Autodesk Inventor part; units mm, degrees
(part 5 of 6)
  line L2000 (-9.6394, -22.1122) -> (-9.6394, -22.3521) construction
  spline S587 degree 2 poles (-9.6394, -22.3521) (-9.6394, -22.5921) (-9.8794, -22.5921) knots 0 0 0 1 1 1
  line L2001 (-9.6394, -22.3521) -> (-9.6394, -22.5921) construction
  line L2002 (-9.6394, -22.5921) -> (-9.8794, -22.5921) construction
  line L2003 (-9.8794, -22.5921) -> (-10.5952, -22.5921)
  spline S588 degree 2 poles (-20.1571, -30.3351) (-19.8611, -30.3351) (-19.4413, -29.9152) (-19.4413, -29.6193) knots 0 0 0 1 2 2 2
  line L2004 (-20.1571, -30.3351) -> (-19.8611, -30.3351) construction
  line L2005 (-19.8611, -30.3351) -> (-19.4413, -29.9152) construction
  line L2006 (-19.4413, -29.9152) -> (-19.4413, -29.6193) construction
  line L2007 (-19.4413, -29.6193) -> (-19.4413, -27.224)
  spline S589 degree 2 poles (-19.4413, -27.224) (-19.4413, -26.928) (-19.8611, -26.5082) (-20.1571, -26.5082) knots 0 0 0 1 2 2 2
  line L2008 (-19.4413, -27.224) -> (-19.4413, -26.928) construction
  line L2009 (-19.4413, -26.928) -> (-19.8611, -26.5082) construction
  line L2010 (-19.8611, -26.5082) -> (-20.1571, -26.5082) construction
  line L2011 (-20.1571, -30.815) -> (-21.5927, -30.815)
  spline S590 degree 2 poles (-21.5927, -30.815) (-21.6886, -30.815) (-21.8326, -30.671) (-21.8326, -30.575) knots 0 0 0 1 2 2 2
  line L2012 (-21.5927, -30.815) -> (-21.6886, -30.815) construction
  line L2013 (-21.6886, -30.815) -> (-21.8326, -30.671) construction
  line L2014 (-21.8326, -30.671) -> (-21.8326, -30.575) construction
  line L2015 (-21.8326, -30.575) -> (-21.8326, -26.2682)
  spline S591 degree 2 poles (-21.8326, -26.2682) (-21.8326, -26.1723) (-21.6886, -26.0283) (-21.5927, -26.0283) knots 0 0 0 1 2 2 2
  line L2016 (-21.8326, -26.2682) -> (-21.8326, -26.1723) construction
  line L2017 (-21.8326, -26.1723) -> (-21.6886, -26.0283) construction
  line L2018 (-21.6886, -26.0283) -> (-21.5927, -26.0283) construction
  line L2019 (-21.5927, -26.0283) -> (-20.1571, -26.0283)
  spline S592 degree 2 poles (-20.1571, -26.0283) (-19.6612, -26.0283) (-18.9614, -26.7321) (-18.9614, -27.224) knots 0 0 0 1 2 2 2
  line L2020 (-20.1571, -26.0283) -> (-19.6612, -26.0283) construction
  line L2021 (-19.6612, -26.0283) -> (-18.9614, -26.7321) construction
  line L2022 (-18.9614, -26.7321) -> (-18.9614, -27.224) construction
  line L2023 (-18.9614, -27.224) -> (-18.9614, -29.6193)
  spline S593 degree 2 poles (-18.9614, -29.6193) (-18.9614, -30.1152) (-19.6612, -30.815) (-20.1571, -30.815) knots 0 0 0 1 2 2 2
  line L2024 (-18.9614, -29.6193) -> (-18.9614, -30.1152) construction
  line L2025 (-18.9614, -30.1152) -> (-19.6612, -30.815) construction
  line L2026 (-19.6612, -30.815) -> (-20.1571, -30.815) construction
  spline S594 degree 2 poles (-22.6464, -34.2509) (-22.4065, -34.2509) (-22.4065, -34.4908) knots 0 0 0 1 1 1
  line L2027 (-22.6464, -34.2509) -> (-22.4065, -34.2509) construction
  line L2028 (-22.4065, -34.2509) -> (-22.4065, -34.4908) construction
  spline S595 degree 2 poles (-22.4065, -34.4908) (-22.4065, -34.7308) (-22.6464, -34.7308) knots 0 0 0 1 1 1
  line L2029 (-22.4065, -34.4908) -> (-22.4065, -34.7308) construction
  line L2030 (-22.4065, -34.7308) -> (-22.6464, -34.7308) construction
  spline S596 degree 2 poles (-24.322, -36.8902) (-24.322, -37.1301) (-24.5619, -37.1301) knots 0 0 0 1 1 1
  line L2031 (-24.322, -36.8902) -> (-24.322, -37.1301) construction
  line L2032 (-24.322, -37.1301) -> (-24.5619, -37.1301) construction
  spline S597 degree 2 poles (-24.5619, -37.1301) (-24.8018, -37.1301) (-24.8018, -36.8902) knots 0 0 0 1 1 1
  line L2033 (-24.5619, -37.1301) -> (-24.8018, -37.1301) construction
  line L2034 (-24.8018, -37.1301) -> (-24.8018, -36.8902) construction
  line L2035 (-24.8018, -36.8902) -> (-24.8018, -32.5834)
  spline S598 degree 2 poles (-24.8018, -32.5834) (-24.8018, -32.3434) (-24.5619, -32.3434) knots 0 0 0 1 1 1
  line L2036 (-24.8018, -32.5834) -> (-24.8018, -32.3434) construction
  line L2037 (-24.8018, -32.3434) -> (-24.5619, -32.3434) construction
  line L2038 (-24.5619, -32.3434) -> (-22.6464, -32.3434)
  spline S599 degree 2 poles (-22.6464, -32.3434) (-22.4065, -32.3434) (-22.4065, -32.5834) knots 0 0 0 1 1 1
  line L2039 (-22.6464, -32.3434) -> (-22.4065, -32.3434) construction
  line L2040 (-22.4065, -32.3434) -> (-22.4065, -32.5834) construction
  spline S600 degree 2 poles (-22.4065, -32.5834) (-22.4065, -32.8233) (-22.6464, -32.8233) knots 0 0 0 1 1 1
  line L2041 (-22.4065, -32.5834) -> (-22.4065, -32.8233) construction
  line L2042 (-22.4065, -32.8233) -> (-22.6464, -32.8233) construction
  line L2043 (10.7293, -22.5371) -> (9.5336, -22.5371)
  spline S601 degree 2 poles (9.5336, -22.5371) (9.1417, -22.5371) (8.5779, -21.9772) (8.5779, -21.5813) knots 0 0 0 1 2 2 2
  line L2044 (9.5336, -22.5371) -> (9.1417, -22.5371) construction
  line L2045 (9.1417, -22.5371) -> (8.5779, -21.9772) construction
  line L2046 (8.5779, -21.9772) -> (8.5779, -21.5813) construction
  line L2047 (8.5779, -21.5813) -> (8.5779, -19.426)
  spline S602 degree 2 poles (8.5779, -19.426) (8.5779, -19.186) (8.8178, -19.186) knots 0 0 0 1 1 1
  line L2048 (8.5779, -19.426) -> (8.5779, -19.186) construction
  line L2049 (8.5779, -19.186) -> (8.8178, -19.186) construction
  spline S603 degree 2 poles (8.8178, -19.186) (9.0578, -19.186) (9.0578, -19.426) knots 0 0 0 1 1 1
  line L2050 (8.8178, -19.186) -> (9.0578, -19.186) construction
  line L2051 (9.0578, -19.186) -> (9.0578, -19.426) construction
  line L2052 (9.0578, -19.426) -> (9.0578, -21.5773)
  spline S604 degree 2 poles (9.0578, -21.5773) (9.0578, -21.7733) (9.3377, -22.0572) (9.5336, -22.0572) knots 0 0 0 1 2 2 2
  line L2053 (9.0578, -21.5773) -> (9.0578, -21.7733) construction
  line L2054 (9.0578, -21.7733) -> (9.3377, -22.0572) construction
  line L2055 (9.3377, -22.0572) -> (9.5336, -22.0572) construction
  spline S605 degree 2 poles (10.4894, -19.426) (10.4894, -19.186) (10.7293, -19.186) knots 0 0 0 1 1 1
  line L2056 (10.4894, -19.426) -> (10.4894, -19.186) construction
  line L2057 (10.4894, -19.186) -> (10.7293, -19.186) construction
  spline S606 degree 2 poles (10.7293, -19.186) (10.9692, -19.186) (10.9692, -19.426) knots 0 0 0 1 1 1
  line L2058 (10.7293, -19.186) -> (10.9692, -19.186) construction
  line L2059 (10.9692, -19.186) -> (10.9692, -19.426) construction
  line L2060 (10.9692, -19.426) -> (10.9692, -22.2971)
  spline S607 degree 2 poles (10.9692, -22.2971) (10.9692, -22.5371) (10.7293, -22.5371) knots 0 0 0 1 1 1
  line L2061 (10.9692, -22.2971) -> (10.9692, -22.5371) construction
  line L2062 (10.9692, -22.5371) -> (10.7293, -22.5371) construction
  spline S608 degree 2 poles (17.6713, -22.5371) (17.4314, -22.5371) (17.4314, -22.2971) knots 0 0 0 1 1 1
  line L2063 (17.6713, -22.5371) -> (17.4314, -22.5371) construction
  line L2064 (17.4314, -22.5371) -> (17.4314, -22.2971) construction
  spline S609 degree 2 poles (16.6716, -21.2374) (16.5797, -21.3694) (16.4757, -21.3694) knots 0 0 0 1 1 1
  line L2065 (16.6716, -21.2374) -> (16.5797, -21.3694) construction
  line L2066 (16.5797, -21.3694) -> (16.4757, -21.3694) construction
  spline S610 degree 2 poles (16.4757, -21.3694) (16.3717, -21.3694) (16.2797, -21.2374) knots 0 0 0 1 1 1
  line L2067 (16.4757, -21.3694) -> (16.3717, -21.3694) construction
  line L2068 (16.3717, -21.3694) -> (16.2797, -21.2374) construction
  spline S611 degree 2 poles (15.52, -22.2971) (15.52, -22.5371) (15.28, -22.5371) knots 0 0 0 1 1 1
  line L2069 (15.52, -22.2971) -> (15.52, -22.5371) construction
  line L2070 (15.52, -22.5371) -> (15.28, -22.5371) construction
  spline S612 degree 2 poles (15.28, -22.5371) (15.0401, -22.5371) (15.0401, -22.2971) knots 0 0 0 1 1 1
  line L2071 (15.28, -22.5371) -> (15.0401, -22.5371) construction
  line L2072 (15.0401, -22.5371) -> (15.0401, -22.2971) construction
  line L2073 (15.0401, -22.2971) -> (15.0401, -19.422)
  spline S613 degree 2 poles (15.0401, -19.422) (15.0401, -19.146) (15.252, -19.146) knots 0 0 0 1 1 1
  line L2074 (15.0401, -19.422) -> (15.0401, -19.146) construction
  line L2075 (15.0401, -19.146) -> (15.252, -19.146) construction
  spline S614 degree 2 poles (15.252, -19.146) (15.376, -19.146) (15.476, -19.286) knots 0 0 0 1 1 1
  line L2076 (15.252, -19.146) -> (15.376, -19.146) construction
  line L2077 (15.376, -19.146) -> (15.476, -19.286) construction
  spline S615 degree 2 poles (17.4754, -19.286) (17.5754, -19.146) (17.6993, -19.146) knots 0 0 0 1 1 1
  line L2078 (17.4754, -19.286) -> (17.5754, -19.146) construction
  line L2079 (17.5754, -19.146) -> (17.6993, -19.146) construction
  spline S616 degree 2 poles (17.6993, -19.146) (17.9113, -19.146) (17.9113, -19.422) knots 0 0 0 1 1 1
  line L2080 (17.6993, -19.146) -> (17.9113, -19.146) construction
  line L2081 (17.9113, -19.146) -> (17.9113, -19.422) construction
  line L2082 (17.9113, -19.422) -> (17.9113, -22.2971)
  spline S617 degree 2 poles (17.9113, -22.2971) (17.9113, -22.5371) (17.6713, -22.5371) knots 0 0 0 1 1 1
  line L2083 (17.9113, -22.2971) -> (17.9113, -22.5371) construction
  line L2084 (17.9113, -22.5371) -> (17.6713, -22.5371) construction
  spline S618 degree 2 poles (7.7252, -27.8713) (7.9211, -27.8713) (8.2011, -27.5874) (8.2011, -27.3914) knots 0 0 0 1 2 2 2
  line L2085 (7.7252, -27.8713) -> (7.9211, -27.8713) construction
  line L2086 (7.9211, -27.8713) -> (8.2011, -27.5874) construction
  line L2087 (8.2011, -27.5874) -> (8.2011, -27.3914) construction
  line L2088 (8.2011, -27.3914) -> (8.2011, -25.9598)
  spline S619 degree 2 poles (8.2011, -25.9598) (8.2011, -25.7639) (7.9211, -25.48) (7.7252, -25.48) knots 0 0 0 1 2 2 2
  line L2089 (8.2011, -25.9598) -> (8.2011, -25.7639) construction
  line L2090 (8.2011, -25.7639) -> (7.9211, -25.48) construction
  line L2091 (7.9211, -25.48) -> (7.7252, -25.48) construction
  line L2092 (7.7252, -25.48) -> (7.2453, -25.48)
  spline S620 degree 2 poles (7.2453, -25.48) (7.0494, -25.48) (6.7695, -25.7639) (6.7695, -25.9598) knots 0 0 0 1 2 2 2
  line L2093 (7.2453, -25.48) -> (7.0494, -25.48) construction
  line L2094 (7.0494, -25.48) -> (6.7695, -25.7639) construction
  line L2095 (6.7695, -25.7639) -> (6.7695, -25.9598) construction
  line L2096 (6.7695, -25.9598) -> (6.7695, -27.3914)
  spline S621 degree 2 poles (6.7695, -27.3914) (6.7695, -27.5874) (7.0494, -27.8713) (7.2453, -27.8713) knots 0 0 0 1 2 2 2
  line L2097 (6.7695, -27.3914) -> (6.7695, -27.5874) construction
  line L2098 (6.7695, -27.5874) -> (7.0494, -27.8713) construction
  line L2099 (7.0494, -27.8713) -> (7.2453, -27.8713) construction
  line L2100 (7.2453, -27.8713) -> (7.7252, -27.8713)
  spline S622 degree 2 poles (6.3616, -23.9764) (6.2736, -23.8884) (6.2736, -23.7804) knots 0 0 0 1 1 1
  line L2101 (6.3616, -23.9764) -> (6.2736, -23.8884) construction
  line L2102 (6.2736, -23.8884) -> (6.2736, -23.7804) construction
  spline S623 degree 2 poles (6.2736, -23.7804) (6.2736, -23.5645) (6.5255, -23.5645) knots 0 0 0 1 1 1
  line L2103 (6.2736, -23.7804) -> (6.2736, -23.5645) construction
  line L2104 (6.2736, -23.5645) -> (6.5255, -23.5645) construction
  line L2105 (6.5255, -23.5645) -> (8.441, -23.5645)
  spline S624 degree 2 poles (8.441, -23.5645) (8.6809, -23.5645) (8.6809, -23.8044) knots 0 0 0 1 1 1
  line L2106 (8.441, -23.5645) -> (8.6809, -23.5645) construction
  line L2107 (8.6809, -23.5645) -> (8.6809, -23.8044) construction
  spline S625 degree 2 poles (8.6809, -23.8044) (8.6809, -24.0444) (8.441, -24.0444) knots 0 0 0 1 1 1
  line L2108 (8.6809, -23.8044) -> (8.6809, -24.0444) construction
  line L2109 (8.6809, -24.0444) -> (8.441, -24.0444) construction
  spline S626 degree 2 poles (8.393, -25.256) (8.433, -25.288) (8.453, -25.332) knots 0 0 0 1 1 1
  line L2110 (8.393, -25.256) -> (8.433, -25.288) construction
  line L2111 (8.433, -25.288) -> (8.453, -25.332) construction
  spline S627 degree 2 poles (8.453, -25.332) (8.6809, -25.5999) (8.6809, -25.9598) knots 0 0 0 1 1 1
  line L2112 (8.453, -25.332) -> (8.6809, -25.5999) construction
  line L2113 (8.6809, -25.5999) -> (8.6809, -25.9598) construction
  line L2114 (8.6809, -25.9598) -> (8.6809, -27.3954)
  spline S628 degree 2 poles (8.6809, -27.3954) (8.6809, -27.7913) (8.1211, -28.3512) (7.7252, -28.3512) knots 0 0 0 1 2 2 2
  line L2115 (8.6809, -27.3954) -> (8.6809, -27.7913) construction
  line L2116 (8.6809, -27.7913) -> (8.1211, -28.3512) construction
  line L2117 (8.1211, -28.3512) -> (7.7252, -28.3512) construction
  line L2118 (7.7252, -28.3512) -> (7.2453, -28.3512)
  spline S629 degree 2 poles (7.2453, -28.3512) (6.8534, -28.3512) (6.2896, -27.7913) (6.2896, -27.3954) knots 0 0 0 1 2 2 2
  line L2119 (7.2453, -28.3512) -> (6.8534, -28.3512) construction
  line L2120 (6.8534, -28.3512) -> (6.2896, -27.7913) construction
  line L2121 (6.2896, -27.7913) -> (6.2896, -27.3954) construction
  line L2122 (6.2896, -27.3954) -> (6.2896, -25.9558)
  spline S630 degree 2 poles (6.2896, -25.9558) (6.2896, -25.5599) (6.8534, -25.0001) (7.2453, -25.0001) knots 0 0 0 1 2 2 2
  line L2123 (6.2896, -25.9558) -> (6.2896, -25.5599) construction
  line L2124 (6.2896, -25.5599) -> (6.8534, -25.0001) construction
  line L2125 (6.8534, -25.0001) -> (7.2453, -25.0001) construction
  spline S631 degree 2 poles (11.0763, -27.8713) (11.2722, -27.8713) (11.5521, -27.5874) (11.5521, -27.3914) knots 0 0 0 1 2 2 2
  line L2126 (11.0763, -27.8713) -> (11.2722, -27.8713) construction
  line L2127 (11.2722, -27.8713) -> (11.5521, -27.5874) construction
  line L2128 (11.5521, -27.5874) -> (11.5521, -27.3914) construction
  spline S632 degree 2 poles (10.5964, -25.48) (10.4004, -25.48) (10.1205, -25.7639) (10.1205, -25.9598) knots 0 0 0 1 2 2 2
  line L2129 (10.5964, -25.48) -> (10.4004, -25.48) construction
  line L2130 (10.4004, -25.48) -> (10.1205, -25.7639) construction
  line L2131 (10.1205, -25.7639) -> (10.1205, -25.9598) construction
  line L2132 (10.1205, -25.9598) -> (10.1205, -27.3914)
  spline S633 degree 2 poles (10.1205, -27.3914) (10.1205, -27.5874) (10.4004, -27.8713) (10.5964, -27.8713) knots 0 0 0 1 2 2 2
  line L2133 (10.1205, -27.3914) -> (10.1205, -27.5874) construction
  line L2134 (10.1205, -27.5874) -> (10.4004, -27.8713) construction
  line L2135 (10.4004, -27.8713) -> (10.5964, -27.8713) construction
  line L2136 (10.5964, -27.8713) -> (11.0763, -27.8713)
  line L2137 (11.0763, -28.3512) -> (10.5964, -28.3512)
  spline S634 degree 2 poles (10.5964, -28.3512) (10.2045, -28.3512) (9.6407, -27.7913) (9.6407, -27.3954) knots 0 0 0 1 2 2 2
  line L2138 (10.5964, -28.3512) -> (10.2045, -28.3512) construction
  line L2139 (10.2045, -28.3512) -> (9.6407, -27.7913) construction
  line L2140 (9.6407, -27.7913) -> (9.6407, -27.3954) construction
  line L2141 (9.6407, -27.3954) -> (9.6407, -25.9558)
  spline S635 degree 2 poles (9.6407, -25.9558) (9.6407, -25.5599) (10.2045, -25.0001) (10.5964, -25.0001) knots 0 0 0 1 2 2 2
  line L2142 (9.6407, -25.9558) -> (9.6407, -25.5599) construction
  line L2143 (9.6407, -25.5599) -> (10.2045, -25.0001) construction
  line L2144 (10.2045, -25.0001) -> (10.5964, -25.0001) construction
  line L2145 (10.5964, -25.0001) -> (11.7921, -25.0001)
  spline S636 degree 2 poles (11.7921, -25.0001) (12.032, -25.0001) (12.032, -25.24) knots 0 0 0 1 1 1
  line L2146 (11.7921, -25.0001) -> (12.032, -25.0001) construction
  line L2147 (12.032, -25.0001) -> (12.032, -25.24) construction
  line L2148 (12.032, -25.24) -> (12.032, -27.3874)
  spline S637 degree 2 poles (12.032, -27.3874) (12.032, -27.7473) (12.3679, -27.8913) knots 0 0 0 1 1 1
  line L2149 (12.032, -27.3874) -> (12.032, -27.7473) construction
  line L2150 (12.032, -27.7473) -> (12.3679, -27.8913) construction
  spline S638 degree 2 poles (12.3679, -27.8913) (12.5159, -27.9513) (12.5159, -28.1032) knots 0 0 0 1 1 1
  line L2151 (12.3679, -27.8913) -> (12.5159, -27.9513) construction
  line L2152 (12.5159, -27.9513) -> (12.5159, -28.1032) construction
  spline S639 degree 2 poles (12.5159, -28.1032) (12.5159, -28.2032) (12.3799, -28.3552) (12.2799, -28.3552) knots 0 0 0 1 2 2 2
  line L2153 (12.5159, -28.1032) -> (12.5159, -28.2032) construction
  line L2154 (12.5159, -28.2032) -> (12.3799, -28.3552) construction
  line L2155 (12.3799, -28.3552) -> (12.2799, -28.3552) construction
  spline S640 degree 2 poles (12.2799, -28.3552) (12.2279, -28.3552) (12.1759, -28.3312) knots 0 0 0 1 1 1
  line L2156 (12.2799, -28.3552) -> (12.2279, -28.3552) construction
  line L2157 (12.2279, -28.3552) -> (12.1759, -28.3312) construction
  spline S641 degree 2 poles (12.1759, -28.3312) (11.936, -28.2272) (11.7881, -28.0352) knots 0 0 0 1 1 1
  line L2158 (12.1759, -28.3312) -> (11.936, -28.2272) construction
  line L2159 (11.936, -28.2272) -> (11.7881, -28.0352) construction
  spline S642 degree 2 poles (11.7881, -28.0352) (11.5001, -28.3512) (11.0763, -28.3512) knots 0 0 0 1 1 1
  line L2160 (11.7881, -28.0352) -> (11.5001, -28.3512) construction
  line L2161 (11.5001, -28.3512) -> (11.0763, -28.3512) construction
  spline S643 degree 2 poles (14.4273, -27.8713) (14.6233, -27.8713) (14.9032, -27.5874) (14.9032, -27.3914) knots 0 0 0 1 2 2 2
  line L2162 (14.4273, -27.8713) -> (14.6233, -27.8713) construction
  line L2163 (14.6233, -27.8713) -> (14.9032, -27.5874) construction
  line L2164 (14.9032, -27.5874) -> (14.9032, -27.3914) construction
  line L2165 (14.9032, -27.3914) -> (14.9032, -25.9598)
  spline S644 degree 2 poles (14.9032, -25.9598) (14.9032, -25.7639) (14.6233, -25.48) (14.4273, -25.48) knots 0 0 0 1 2 2 2
  line L2166 (14.9032, -25.9598) -> (14.9032, -25.7639) construction
  line L2167 (14.9032, -25.7639) -> (14.6233, -25.48) construction
  line L2168 (14.6233, -25.48) -> (14.4273, -25.48) construction
  spline S645 degree 2 poles (13.4716, -29.5468) (13.4716, -29.7867) (13.2317, -29.7867) knots 0 0 0 1 1 1
  line L2169 (13.4716, -29.5468) -> (13.4716, -29.7867) construction
  line L2170 (13.4716, -29.7867) -> (13.2317, -29.7867) construction
  spline S646 degree 2 poles (13.2317, -29.7867) (12.9917, -29.7867) (12.9917, -29.5468) knots 0 0 0 1 1 1
  line L2171 (13.2317, -29.7867) -> (12.9917, -29.7867) construction
  line L2172 (12.9917, -29.7867) -> (12.9917, -29.5468) construction
  line L2173 (12.9917, -29.5468) -> (12.9917, -25.24)
  spline S647 degree 2 poles (12.9917, -25.24) (12.9917, -25.0001) (13.2317, -25.0001) knots 0 0 0 1 1 1
  line L2174 (12.9917, -25.24) -> (12.9917, -25.0001) construction
  line L2175 (12.9917, -25.0001) -> (13.2317, -25.0001) construction
  line L2176 (13.2317, -25.0001) -> (14.4273, -25.0001)
  spline S648 degree 2 poles (14.4273, -25.0001) (14.8232, -25.0001) (15.383, -25.5599) (15.383, -25.9558) knots 0 0 0 1 2 2 2
  line L2177 (14.4273, -25.0001) -> (14.8232, -25.0001) construction
  line L2178 (14.8232, -25.0001) -> (15.383, -25.5599) construction
  line L2179 (15.383, -25.5599) -> (15.383, -25.9558) construction
  line L2180 (15.383, -25.9558) -> (15.383, -27.3954)
  spline S649 degree 2 poles (15.383, -27.3954) (15.383, -27.7913) (14.8232, -28.3512) (14.4273, -28.3512) knots 0 0 0 1 2 2 2
  line L2181 (15.383, -27.3954) -> (15.383, -27.7913) construction
  line L2182 (15.383, -27.7913) -> (14.8232, -28.3512) construction
  line L2183 (14.8232, -28.3512) -> (14.4273, -28.3512) construction
  spline S650 degree 2 poles (7.6622, -35.058) (7.8581, -35.058) (8.138, -34.7741) (8.138, -34.5782) knots 0 0 0 1 2 2 2
  line L2184 (7.6622, -35.058) -> (7.8581, -35.058) construction
  line L2185 (7.8581, -35.058) -> (8.138, -34.7741) construction
  line L2186 (8.138, -34.7741) -> (8.138, -34.5782) construction
  spline S651 degree 2 poles (7.1823, -32.6667) (6.9863, -32.6667) (6.7064, -32.9506) (6.7064, -33.1466) knots 0 0 0 1 2 2 2
  line L2187 (7.1823, -32.6667) -> (6.9863, -32.6667) construction
  line L2188 (6.9863, -32.6667) -> (6.7064, -32.9506) construction
  line L2189 (6.7064, -32.9506) -> (6.7064, -33.1466) construction
  line L2190 (6.7064, -33.1466) -> (6.7064, -34.5782)
  spline S652 degree 2 poles (6.7064, -34.5782) (6.7064, -34.7741) (6.9863, -35.058) (7.1823, -35.058) knots 0 0 0 1 2 2 2
  line L2191 (6.7064, -34.5782) -> (6.7064, -34.7741) construction
  line L2192 (6.7064, -34.7741) -> (6.9863, -35.058) construction
  line L2193 (6.9863, -35.058) -> (7.1823, -35.058) construction
  line L2194 (7.1823, -35.058) -> (7.6622, -35.058)
  line L2195 (7.6622, -35.5379) -> (7.1823, -35.5379)
  spline S653 degree 2 poles (7.1823, -35.5379) (6.7904, -35.5379) (6.2266, -34.9781) (6.2266, -34.5822) knots 0 0 0 1 2 2 2
  line L2196 (7.1823, -35.5379) -> (6.7904, -35.5379) construction
  line L2197 (6.7904, -35.5379) -> (6.2266, -34.9781) construction
  line L2198 (6.2266, -34.9781) -> (6.2266, -34.5822) construction
  line L2199 (6.2266, -34.5822) -> (6.2266, -33.1426)
  spline S654 degree 2 poles (6.2266, -33.1426) (6.2266, -32.7467) (6.7904, -32.1868) (7.1823, -32.1868) knots 0 0 0 1 2 2 2
  line L2200 (6.2266, -33.1426) -> (6.2266, -32.7467) construction
  line L2201 (6.2266, -32.7467) -> (6.7904, -32.1868) construction
  line L2202 (6.7904, -32.1868) -> (7.1823, -32.1868) construction
  line L2203 (7.1823, -32.1868) -> (8.3779, -32.1868)
  spline S655 degree 2 poles (8.3779, -32.1868) (8.6179, -32.1868) (8.6179, -32.4268) knots 0 0 0 1 1 1
  line L2204 (8.3779, -32.1868) -> (8.6179, -32.1868) construction
  line L2205 (8.6179, -32.1868) -> (8.6179, -32.4268) construction
  line L2206 (8.6179, -32.4268) -> (8.6179, -34.5742)
  spline S656 degree 2 poles (8.6179, -34.5742) (8.6179, -34.9341) (8.9538, -35.078) knots 0 0 0 1 1 1
  line L2207 (8.6179, -34.5742) -> (8.6179, -34.9341) construction
  line L2208 (8.6179, -34.9341) -> (8.9538, -35.078) construction
  spline S657 degree 2 poles (8.9538, -35.078) (9.1017, -35.138) (9.1017, -35.29) knots 0 0 0 1 1 1
  line L2209 (8.9538, -35.078) -> (9.1017, -35.138) construction
  line L2210 (9.1017, -35.138) -> (9.1017, -35.29) construction
  spline S658 degree 2 poles (9.1017, -35.29) (9.1017, -35.3899) (8.9658, -35.5419) (8.8658, -35.5419) knots 0 0 0 1 2 2 2
  line L2211 (9.1017, -35.29) -> (9.1017, -35.3899) construction
  line L2212 (9.1017, -35.3899) -> (8.9658, -35.5419) construction
  line L2213 (8.9658, -35.5419) -> (8.8658, -35.5419) construction
  spline S659 degree 2 poles (8.8658, -35.5419) (8.8138, -35.5419) (8.7618, -35.5179) knots 0 0 0 1 1 1
  line L2214 (8.8658, -35.5419) -> (8.8138, -35.5419) construction
  line L2215 (8.8138, -35.5419) -> (8.7618, -35.5179) construction
  spline S660 degree 2 poles (8.7618, -35.5179) (8.5219, -35.4139) (8.374, -35.222) knots 0 0 0 1 1 1
  line L2216 (8.7618, -35.5179) -> (8.5219, -35.4139) construction
  line L2217 (8.5219, -35.4139) -> (8.374, -35.222) construction
  spline S661 degree 2 poles (8.374, -35.222) (8.086, -35.5379) (7.6622, -35.5379) knots 0 0 0 1 1 1
  line L2218 (8.374, -35.222) -> (8.086, -35.5379) construction
  line L2219 (8.086, -35.5379) -> (7.6622, -35.5379) construction
  line L2220 (10.0095, -34.5342) -> (10.0095, -35.298)
  spline S662 degree 2 poles (10.0095, -35.298) (10.0095, -35.5379) (9.7696, -35.5379) knots 0 0 0 1 1 1
  line L2221 (10.0095, -35.298) -> (10.0095, -35.5379) construction
  line L2222 (10.0095, -35.5379) -> (9.7696, -35.5379) construction
  spline S663 degree 2 poles (9.7696, -35.5379) (9.5296, -35.5379) (9.5296, -35.298) knots 0 0 0 1 1 1
  line L2223 (9.7696, -35.5379) -> (9.5296, -35.5379) construction
  line L2224 (9.5296, -35.5379) -> (9.5296, -35.298) construction
  line L2225 (9.5296, -35.298) -> (9.5296, -32.4268)
  spline S664 degree 2 poles (9.5296, -32.4268) (9.5296, -32.1868) (9.7696, -32.1868) knots 0 0 0 1 1 1
  line L2226 (9.5296, -32.4268) -> (9.5296, -32.1868) construction
  line L2227 (9.5296, -32.1868) -> (9.7696, -32.1868) construction
  spline S665 degree 2 poles (9.7696, -32.1868) (10.0095, -32.1868) (10.0095, -32.4268) knots 0 0 0 1 1 1
  line L2228 (9.7696, -32.1868) -> (10.0095, -32.1868) construction
  line L2229 (10.0095, -32.1868) -> (10.0095, -32.4268) construction
  spline S666 degree 2 poles (11.5291, -32.2428) (11.593, -32.1708) (11.681, -32.1708) knots 0 0 0 1 1 1
  line L2230 (11.5291, -32.2428) -> (11.593, -32.1708) construction
  line L2231 (11.593, -32.1708) -> (11.681, -32.1708) construction
  spline S667 degree 2 poles (11.681, -32.1708) (11.777, -32.1708) (11.921, -32.3268) (11.921, -32.4308) knots 0 0 0 1 2 2 2
  line L2232 (11.681, -32.1708) -> (11.777, -32.1708) construction
  line L2233 (11.777, -32.1708) -> (11.921, -32.3268) construction
  line L2234 (11.921, -32.3268) -> (11.921, -32.4308) construction
  spline S668 degree 2 poles (11.921, -32.4308) (11.921, -32.5307) (11.845, -32.6067) knots 0 0 0 1 1 1
  line L2235 (11.921, -32.4308) -> (11.921, -32.5307) construction
  line L2236 (11.921, -32.5307) -> (11.845, -32.6067) construction
  spline S669 degree 2 poles (11.869, -35.142) (11.921, -35.222) (11.921, -35.302) knots 0 0 0 1 1 1
  line L2237 (11.869, -35.142) -> (11.921, -35.222) construction
  line L2238 (11.921, -35.222) -> (11.921, -35.302) construction
  spline S670 degree 2 poles (11.921, -35.302) (11.921, -35.4019) (11.765, -35.5459) (11.677, -35.5459) knots 0 0 0 1 2 2 2
  line L2239 (11.921, -35.302) -> (11.921, -35.4019) construction
  line L2240 (11.921, -35.4019) -> (11.765, -35.5459) construction
  line L2241 (11.765, -35.5459) -> (11.677, -35.5459) construction
  spline S671 degree 2 poles (11.677, -35.5459) (11.5651, -35.5459) (11.5051, -35.4499) knots 0 0 0 1 1 1
  line L2242 (11.677, -35.5459) -> (11.5651, -35.5459) construction
  line L2243 (11.5651, -35.5459) -> (11.5051, -35.4499) construction
  line L2244 (11.5051, -35.4499) -> (10.5453, -33.9703)
  spline S672 degree 2 poles (10.5453, -33.9703) (10.4014, -34.1223) (10.0095, -34.5342) knots 0 0 0 1 1 1
  line L2245 (10.5453, -33.9703) -> (10.4014, -34.1223) construction
  line L2246 (10.4014, -34.1223) -> (10.0095, -34.5342) construction
  spline S673 degree 2 poles (-21.2583, -43.6884) (-21.2583, -43.4485) (-21.0184, -43.4485) knots 0 0 0 1 1 1
  line L2247 (-21.2583, -43.6884) -> (-21.2583, -43.4485) construction
  line L2248 (-21.2583, -43.4485) -> (-21.0184, -43.4485) construction
  spline S674 degree 2 poles (-21.0184, -43.4485) (-20.7785, -43.4485) (-20.7785, -43.6884) knots 0 0 0 1 1 1
  line L2249 (-21.0184, -43.4485) -> (-20.7785, -43.4485) construction
  line L2250 (-20.7785, -43.4485) -> (-20.7785, -43.6884) construction
  line L2251 (-20.7785, -43.6884) -> (-20.7785, -46.5596)
  spline S675 degree 2 poles (-20.7785, -46.5596) (-20.7785, -46.7995) (-21.0184, -46.7995) knots 0 0 0 1 1 1
  line L2252 (-20.7785, -46.5596) -> (-20.7785, -46.7995) construction
  line L2253 (-20.7785, -46.7995) -> (-21.0184, -46.7995) construction
  spline S676 degree 2 poles (-21.0184, -46.7995) (-21.2583, -46.7995) (-21.2583, -46.5596) knots 0 0 0 1 1 1
  line L2254 (-21.0184, -46.7995) -> (-21.2583, -46.7995) construction
  line L2255 (-21.2583, -46.7995) -> (-21.2583, -46.5596) construction
  spline S677 degree 2 poles (-22.6899, -46.5596) (-22.6899, -46.7995) (-22.9299, -46.7995) knots 0 0 0 1 1 1
  line L2256 (-22.6899, -46.5596) -> (-22.6899, -46.7995) construction
  line L2257 (-22.6899, -46.7995) -> (-22.9299, -46.7995) construction
  spline S678 degree 2 poles (-22.9299, -46.7995) (-23.1698, -46.7995) (-23.1698, -46.5596) knots 0 0 0 1 1 1
  line L2258 (-22.9299, -46.7995) -> (-23.1698, -46.7995) construction
  line L2259 (-23.1698, -46.7995) -> (-23.1698, -46.5596) construction
  line L2260 (-23.1698, -46.5596) -> (-23.1698, -43.6884)
  spline S679 degree 2 poles (-23.1698, -43.6884) (-23.1698, -43.4485) (-22.9299, -43.4485) knots 0 0 0 1 1 1
  line L2261 (-23.1698, -43.6884) -> (-23.1698, -43.4485) construction
  line L2262 (-23.1698, -43.4485) -> (-22.9299, -43.4485) construction
  spline S680 degree 2 poles (-22.9299, -43.4485) (-22.6899, -43.4485) (-22.6899, -43.6884) knots 0 0 0 1 1 1
  line L2263 (-22.9299, -43.4485) -> (-22.6899, -43.4485) construction
  line L2264 (-22.6899, -43.4485) -> (-22.6899, -43.6884) construction
  spline S681 degree 2 poles (-11.681, -46.3197) (-11.4851, -46.3197) (-11.2052, -46.0357) (-11.2052, -45.8398) knots 0 0 0 1 2 2 2
  line L2265 (-11.681, -46.3197) -> (-11.4851, -46.3197) construction
  line L2266 (-11.4851, -46.3197) -> (-11.2052, -46.0357) construction
  line L2267 (-11.2052, -46.0357) -> (-11.2052, -45.8398) construction
  line L2268 (-11.2052, -45.8398) -> (-11.2052, -44.4082)
  spline S682 degree 2 poles (-11.2052, -44.4082) (-11.2052, -44.2123) (-11.4851, -43.9283) (-11.681, -43.9283) knots 0 0 0 1 2 2 2
  line L2269 (-11.2052, -44.4082) -> (-11.2052, -44.2123) construction
  line L2270 (-11.2052, -44.2123) -> (-11.4851, -43.9283) construction
  line L2271 (-11.4851, -43.9283) -> (-11.681, -43.9283) construction
  spline S683 degree 2 poles (-12.6368, -47.9952) (-12.6368, -48.2351) (-12.8767, -48.2351) knots 0 0 0 1 1 1
  line L2272 (-12.6368, -47.9952) -> (-12.6368, -48.2351) construction
  line L2273 (-12.6368, -48.2351) -> (-12.8767, -48.2351) construction
  spline S684 degree 2 poles (-12.8767, -48.2351) (-13.1166, -48.2351) (-13.1166, -47.9952) knots 0 0 0 1 1 1
  line L2274 (-12.8767, -48.2351) -> (-13.1166, -48.2351) construction
  line L2275 (-13.1166, -48.2351) -> (-13.1166, -47.9952) construction
  line L2276 (-13.1166, -47.9952) -> (-13.1166, -43.6884)
  spline S685 degree 2 poles (-13.1166, -43.6884) (-13.1166, -43.4485) (-12.8767, -43.4485) knots 0 0 0 1 1 1
  line L2277 (-13.1166, -43.6884) -> (-13.1166, -43.4485) construction
  line L2278 (-13.1166, -43.4485) -> (-12.8767, -43.4485) construction
  line L2279 (-12.8767, -43.4485) -> (-11.681, -43.4485)
  spline S686 degree 2 poles (-11.681, -43.4485) (-11.2852, -43.4485) (-10.7253, -44.0083) (-10.7253, -44.4042) knots 0 0 0 1 2 2 2
  line L2280 (-11.681, -43.4485) -> (-11.2852, -43.4485) construction
  line L2281 (-11.2852, -43.4485) -> (-10.7253, -44.0083) construction
  line L2282 (-10.7253, -44.0083) -> (-10.7253, -44.4042) construction
  line L2283 (-10.7253, -44.4042) -> (-10.7253, -45.8438)
  spline S687 degree 2 poles (-10.7253, -45.8438) (-10.7253, -46.2397) (-11.2852, -46.7995) (-11.681, -46.7995) knots 0 0 0 1 2 2 2
  line L2284 (-10.7253, -45.8438) -> (-10.7253, -46.2397) construction
  line L2285 (-10.7253, -46.2397) -> (-11.2852, -46.7995) construction
  line L2286 (-11.2852, -46.7995) -> (-11.681, -46.7995) construction
  spline S688 degree 2 poles (-8.33, -46.3197) (-8.134, -46.3197) (-7.8541, -46.0357) (-7.8541, -45.8398) knots 0 0 0 1 2 2 2
  line L2287 (-8.33, -46.3197) -> (-8.134, -46.3197) construction
  line L2288 (-8.134, -46.3197) -> (-7.8541, -46.0357) construction
  line L2289 (-7.8541, -46.0357) -> (-7.8541, -45.8398) construction
  spline S689 degree 2 poles (-8.8099, -43.9283) (-9.0058, -43.9283) (-9.2857, -44.2123) (-9.2857, -44.4082) knots 0 0 0 1 2 2 2
  line L2290 (-8.8099, -43.9283) -> (-9.0058, -43.9283) construction
  line L2291 (-9.0058, -43.9283) -> (-9.2857, -44.2123) construction
  line L2292 (-9.2857, -44.2123) -> (-9.2857, -44.4082) construction
  line L2293 (-9.2857, -44.4082) -> (-9.2857, -45.8398)
  spline S690 degree 2 poles (-9.2857, -45.8398) (-9.2857, -46.0357) (-9.0058, -46.3197) (-8.8099, -46.3197) knots 0 0 0 1 2 2 2
  line L2294 (-9.2857, -45.8398) -> (-9.2857, -46.0357) construction
  line L2295 (-9.2857, -46.0357) -> (-9.0058, -46.3197) construction
  line L2296 (-9.0058, -46.3197) -> (-8.8099, -46.3197) construction
  line L2297 (-8.8099, -46.3197) -> (-8.33, -46.3197)
  line L2298 (-8.33, -46.7995) -> (-8.8099, -46.7995)
  spline S691 degree 2 poles (-8.8099, -46.7995) (-9.2017, -46.7995) (-9.7656, -46.2397) (-9.7656, -45.8438) knots 0 0 0 1 2 2 2
  line L2299 (-8.8099, -46.7995) -> (-9.2017, -46.7995) construction
  line L2300 (-9.2017, -46.7995) -> (-9.7656, -46.2397) construction
  line L2301 (-9.7656, -46.2397) -> (-9.7656, -45.8438) construction
  line L2302 (-9.7656, -45.8438) -> (-9.7656, -44.4042)
  spline S692 degree 2 poles (-9.7656, -44.4042) (-9.7656, -44.0083) (-9.2017, -43.4485) (-8.8099, -43.4485) knots 0 0 0 1 2 2 2
  line L2303 (-9.7656, -44.4042) -> (-9.7656, -44.0083) construction
  line L2304 (-9.7656, -44.0083) -> (-9.2017, -43.4485) construction
  line L2305 (-9.2017, -43.4485) -> (-8.8099, -43.4485) construction
  line L2306 (-8.8099, -43.4485) -> (-7.6142, -43.4485)
  spline S693 degree 2 poles (-7.6142, -43.4485) (-7.3743, -43.4485) (-7.3743, -43.6884) knots 0 0 0 1 1 1
  line L2307 (-7.6142, -43.4485) -> (-7.3743, -43.4485) construction
  line L2308 (-7.3743, -43.4485) -> (-7.3743, -43.6884) construction
  line L2309 (-7.3743, -43.6884) -> (-7.3743, -45.8358)
  spline S694 degree 2 poles (-7.3743, -45.8358) (-7.3743, -46.1957) (-7.0384, -46.3397) knots 0 0 0 1 1 1
  line L2310 (-7.3743, -45.8358) -> (-7.3743, -46.1957) construction
  line L2311 (-7.3743, -46.1957) -> (-7.0384, -46.3397) construction
  spline S695 degree 2 poles (-7.0384, -46.3397) (-6.8904, -46.3996) (-6.8904, -46.5516) knots 0 0 0 1 1 1
  line L2312 (-7.0384, -46.3397) -> (-6.8904, -46.3996) construction
  line L2313 (-6.8904, -46.3996) -> (-6.8904, -46.5516) construction
  spline S696 degree 2 poles (-6.8904, -46.5516) (-6.8904, -46.6516) (-7.0264, -46.8035) (-7.1263, -46.8035) knots 0 0 0 1 2 2 2
  line L2314 (-6.8904, -46.5516) -> (-6.8904, -46.6516) construction
  line L2315 (-6.8904, -46.6516) -> (-7.0264, -46.8035) construction
  line L2316 (-7.0264, -46.8035) -> (-7.1263, -46.8035) construction
  spline S697 degree 2 poles (-7.1263, -46.8035) (-7.1783, -46.8035) (-7.2303, -46.7795) knots 0 0 0 1 1 1
  line L2317 (-7.1263, -46.8035) -> (-7.1783, -46.8035) construction
  line L2318 (-7.1783, -46.8035) -> (-7.2303, -46.7795) construction
  spline S698 degree 2 poles (-7.2303, -46.7795) (-7.4702, -46.6756) (-7.6182, -46.4836) knots 0 0 0 1 1 1
  line L2319 (-7.2303, -46.7795) -> (-7.4702, -46.6756) construction
  line L2320 (-7.4702, -46.6756) -> (-7.6182, -46.4836) construction
  spline S699 degree 2 poles (-7.6182, -46.4836) (-7.9061, -46.7995) (-8.33, -46.7995) knots 0 0 0 1 1 1
  line L2321 (-7.6182, -46.4836) -> (-7.9061, -46.7995) construction
  line L2322 (-7.9061, -46.7995) -> (-8.33, -46.7995) construction
  line L2323 (-5.9347, -42.8726) -> (-5.9347, -43.6164)
  spline S700 degree 2 poles (-5.9347, -43.6164) (-5.7467, -43.4965) (-5.4588, -43.2845) knots 0 0 0 1 1 1
  line L2324 (-5.9347, -43.6164) -> (-5.7467, -43.4965) construction
  line L2325 (-5.7467, -43.4965) -> (-5.4588, -43.2845) construction
  spline S701 degree 2 poles (-5.4588, -43.2845) (-5.1709, -43.0526) (-5.1709, -42.8726) knots 0 0 0 1 1 1
  line L2326 (-5.4588, -43.2845) -> (-5.1709, -43.0526) construction
  line L2327 (-5.1709, -43.0526) -> (-5.1709, -42.8726) construction
  spline S702 degree 2 poles (-5.1709, -42.8726) (-5.1709, -42.6887) (-5.2908, -42.5847) knots 0 0 0 1 1 1
  line L2328 (-5.1709, -42.8726) -> (-5.1709, -42.6887) construction
  line L2329 (-5.1709, -42.6887) -> (-5.2908, -42.5847) construction
  spline S703 degree 2 poles (-5.2908, -42.5847) (-5.3988, -42.4927) (-5.5508, -42.4927) knots 0 0 0 1 1 1
  line L2330 (-5.2908, -42.5847) -> (-5.3988, -42.4927) construction
  line L2331 (-5.3988, -42.4927) -> (-5.5508, -42.4927) construction
  spline S704 degree 2 poles (-5.5508, -42.4927) (-5.7107, -42.4927) (-5.8147, -42.5847) knots 0 0 0 1 1 1
  line L2332 (-5.5508, -42.4927) -> (-5.7107, -42.4927) construction
  line L2333 (-5.7107, -42.4927) -> (-5.8147, -42.5847) construction
  spline S705 degree 2 poles (-5.8147, -42.5847) (-5.9347, -42.6887) (-5.9347, -42.8726) knots 0 0 0 1 1 1
  line L2334 (-5.8147, -42.5847) -> (-5.9347, -42.6887) construction
  line L2335 (-5.9347, -42.6887) -> (-5.9347, -42.8726) construction
  spline S706 degree 2 poles (-4.9789, -46.3197) (-4.783, -46.3197) (-4.5031, -46.0357) (-4.5031, -45.8398) knots 0 0 0 1 2 2 2
  line L2336 (-4.9789, -46.3197) -> (-4.783, -46.3197) construction
  line L2337 (-4.783, -46.3197) -> (-4.5031, -46.0357) construction
  line L2338 (-4.5031, -46.0357) -> (-4.5031, -45.8398) construction
  line L2339 (-4.5031, -45.8398) -> (-4.5031, -44.4042)
  spline S707 degree 2 poles (-4.5031, -44.4042) (-4.5031, -44.2083) (-4.783, -43.9243) (-4.9789, -43.9243) knots 0 0 0 1 2 2 2
  line L2340 (-4.5031, -44.4042) -> (-4.5031, -44.2083) construction
  line L2341 (-4.5031, -44.2083) -> (-4.783, -43.9243) construction
  line L2342 (-4.783, -43.9243) -> (-4.9789, -43.9243) construction
  line L2343 (-4.9789, -43.9243) -> (-5.4588, -43.9243)
  spline S708 degree 2 poles (-5.4588, -43.9243) (-5.6547, -43.9243) (-5.9347, -44.2083) (-5.9347, -44.4042) knots 0 0 0 1 2 2 2
  line L2344 (-5.4588, -43.9243) -> (-5.6547, -43.9243) construction
  line L2345 (-5.6547, -43.9243) -> (-5.9347, -44.2083) construction
  line L2346 (-5.9347, -44.2083) -> (-5.9347, -44.4042) construction
  line L2347 (-5.9347, -44.4042) -> (-5.9347, -45.8398)
  spline S709 degree 2 poles (-5.9347, -45.8398) (-5.9347, -46.0357) (-5.6547, -46.3197) (-5.4588, -46.3197) knots 0 0 0 1 2 2 2
  line L2348 (-5.9347, -45.8398) -> (-5.9347, -46.0357) construction
  line L2349 (-5.9347, -46.0357) -> (-5.6547, -46.3197) construction
  line L2350 (-5.6547, -46.3197) -> (-5.4588, -46.3197) construction
  line L2351 (-5.4588, -46.3197) -> (-4.9789, -46.3197)
  spline S710 degree 2 poles (-4.2591, -43.7364) (-4.0232, -43.9883) (-4.0232, -44.4042) knots 0 0 0 1 1 1
  line L2352 (-4.2591, -43.7364) -> (-4.0232, -43.9883) construction
  line L2353 (-4.0232, -43.9883) -> (-4.0232, -44.4042) construction
  line L2354 (-4.0232, -44.4042) -> (-4.0232, -45.8438)
  spline S711 degree 2 poles (-4.0232, -45.8438) (-4.0232, -46.2397) (-4.583, -46.7995) (-4.9789, -46.7995) knots 0 0 0 1 2 2 2
  line L2355 (-4.0232, -45.8438) -> (-4.0232, -46.2397) construction
  line L2356 (-4.0232, -46.2397) -> (-4.583, -46.7995) construction
  line L2357 (-4.583, -46.7995) -> (-4.9789, -46.7995) construction
  line L2358 (-4.9789, -46.7995) -> (-5.4588, -46.7995)
  spline S712 degree 2 poles (-5.4588, -46.7995) (-5.8507, -46.7995) (-6.4145, -46.2397) (-6.4145, -45.8438) knots 0 0 0 1 2 2 2
  line L2359 (-5.4588, -46.7995) -> (-5.8507, -46.7995) construction
  line L2360 (-5.8507, -46.7995) -> (-6.4145, -46.2397) construction
  line L2361 (-6.4145, -46.2397) -> (-6.4145, -45.8438) construction
  line L2362 (-6.4145, -45.8438) -> (-6.4145, -42.8726)
  spline S713 degree 2 poles (-6.4145, -42.8726) (-6.4145, -42.4688) (-6.1466, -42.2288) knots 0 0 0 1 1 1
  line L2363 (-6.4145, -42.8726) -> (-6.4145, -42.4688) construction
  line L2364 (-6.4145, -42.4688) -> (-6.1466, -42.2288) construction
  spline S714 degree 2 poles (-6.1466, -42.2288) (-5.9027, -42.0129) (-5.5468, -42.0129) knots 0 0 0 1 1 1
  line L2365 (-6.1466, -42.2288) -> (-5.9027, -42.0129) construction
  line L2366 (-5.9027, -42.0129) -> (-5.5468, -42.0129) construction
  spline S715 degree 2 poles (-5.5468, -42.0129) (-5.1989, -42.0129) (-4.9589, -42.2248) knots 0 0 0 1 1 1
  line L2367 (-5.5468, -42.0129) -> (-5.1989, -42.0129) construction
  line L2368 (-5.1989, -42.0129) -> (-4.9589, -42.2248) construction
  spline S716 degree 2 poles (-4.9589, -42.2248) (-4.691, -42.4648) (-4.691, -42.8686) knots 0 0 0 1 1 1
  line L2369 (-4.9589, -42.2248) -> (-4.691, -42.4648) construction
  line L2370 (-4.691, -42.4648) -> (-4.691, -42.8686) construction
  spline S717 degree 2 poles (-4.691, -42.8686) (-4.691, -43.2725) (-4.9789, -43.4645) knots 0 0 0 1 1 1
  line L2371 (-4.691, -42.8686) -> (-4.691, -43.2725) construction
  line L2372 (-4.691, -43.2725) -> (-4.9789, -43.4645) construction
  spline S718 degree 2 poles (-4.9789, -43.4645) (-4.5151, -43.4645) (-4.2591, -43.7364) knots 0 0 0 1 1 1
  line L2373 (-4.9789, -43.4645) -> (-4.5151, -43.4645) construction
  line L2374 (-4.5151, -43.4645) -> (-4.2591, -43.7364) construction
  spline S719 degree 2 poles (1.2433, -43.9283) (1.0194, -43.9283) (0.7675, -44.2083) (0.7675, -44.4042) knots 0 0 0 1 2 2 2
  line L2375 (1.2433, -43.9283) -> (1.0194, -43.9283) construction
  line L2376 (1.0194, -43.9283) -> (0.7675, -44.2083) construction
  line L2377 (0.7675, -44.2083) -> (0.7675, -44.4042) construction
  spline S720 degree 2 poles (0.7675, -44.4042) (0.7675, -44.6002) (0.8874, -44.7361) knots 0 0 0 1 1 1
  line L2378 (0.7675, -44.4042) -> (0.7675, -44.6002) construction
  line L2379 (0.7675, -44.6002) -> (0.8874, -44.7361) construction
  spline S721 degree 2 poles (0.8874, -44.7361) (1.0194, -44.8841) (1.2433, -44.8841) knots 0 0 0 1 1 1
  line L2380 (0.8874, -44.7361) -> (1.0194, -44.8841) construction
  line L2381 (1.0194, -44.8841) -> (1.2433, -44.8841) construction
  spline S722 degree 2 poles (0.7275, -46.6916) (0.6555, -46.8035) (0.5355, -46.8035) knots 0 0 0 1 1 1
  line L2382 (0.7275, -46.6916) -> (0.6555, -46.8035) construction
  line L2383 (0.6555, -46.8035) -> (0.5355, -46.8035) construction
  spline S723 degree 2 poles (0.5355, -46.8035) (0.4355, -46.8035) (0.2836, -46.6596) (0.2836, -46.5636) knots 0 0 0 1 2 2 2
  line L2384 (0.5355, -46.8035) -> (0.4355, -46.8035) construction
  line L2385 (0.4355, -46.8035) -> (0.2836, -46.6596) construction
  line L2386 (0.2836, -46.6596) -> (0.2836, -46.5636) construction
  spline S724 degree 2 poles (0.2836, -46.5636) (0.2836, -46.4916) (0.3276, -46.4276) knots 0 0 0 1 1 1
  line L2387 (0.2836, -46.5636) -> (0.2836, -46.4916) construction
  line L2388 (0.2836, -46.4916) -> (0.3276, -46.4276) construction
  line L2389 (0.3276, -46.4276) -> (1.0474, -45.3479)
  spline S725 degree 2 poles (1.0474, -45.3479) (0.6875, -45.288) (0.4755, -45.004) knots 0 0 0 1 1 1
  line L2390 (1.0474, -45.3479) -> (0.6875, -45.288) construction
  line L2391 (0.6875, -45.288) -> (0.4755, -45.004) construction
  spline S726 degree 2 poles (0.4755, -45.004) (0.2876, -44.7481) (0.2876, -44.4042) knots 0 0 0 1 1 1
  line L2392 (0.4755, -45.004) -> (0.2876, -44.7481) construction
  line L2393 (0.2876, -44.7481) -> (0.2876, -44.4042) construction
  spline S727 degree 2 poles (0.2876, -44.4042) (0.2876, -44.0163) (0.5275, -43.7484) knots 0 0 0 1 1 1
  line L2394 (0.2876, -44.4042) -> (0.2876, -44.0163) construction
  line L2395 (0.2876, -44.0163) -> (0.5275, -43.7484) construction
  spline S728 degree 2 poles (0.5275, -43.7484) (0.7914, -43.4485) (1.2433, -43.4485) knots 0 0 0 1 1 1
  line L2396 (0.5275, -43.7484) -> (0.7914, -43.4485) construction
  line L2397 (0.7914, -43.4485) -> (1.2433, -43.4485) construction
  line L2398 (1.2433, -43.4485) -> (2.439, -43.4485)
  spline S729 degree 2 poles (2.439, -43.4485) (2.6789, -43.4485) (2.6789, -43.6884) knots 0 0 0 1 1 1
  line L2399 (2.439, -43.4485) -> (2.6789, -43.4485) construction
  line L2400 (2.6789, -43.4485) -> (2.6789, -43.6884) construction
  line L2401 (2.6789, -43.6884) -> (2.6789, -46.5596)
  spline S730 degree 2 poles (2.6789, -46.5596) (2.6789, -46.7995) (2.439, -46.7995) knots 0 0 0 1 1 1
  line L2402 (2.6789, -46.5596) -> (2.6789, -46.7995) construction
  line L2403 (2.6789, -46.7995) -> (2.439, -46.7995) construction
  spline S731 degree 2 poles (2.439, -46.7995) (2.199, -46.7995) (2.199, -46.5596) knots 0 0 0 1 1 1
  line L2404 (2.439, -46.7995) -> (2.199, -46.7995) construction
  line L2405 (2.199, -46.7995) -> (2.199, -46.5596) construction
  spline S732 degree 2 poles (5.6941, -46.3197) (5.834, -46.3197) (6.03, -46.1237) (6.03, -45.9838) knots 0 0 0 1 2 2 2
  line L2406 (5.6941, -46.3197) -> (5.834, -46.3197) construction
  line L2407 (5.834, -46.3197) -> (6.03, -46.1237) construction
  line L2408 (6.03, -46.1237) -> (6.03, -45.9838) construction
  line L2409 (6.03, -45.9838) -> (6.03, -44.2642)
  spline S733 degree 2 poles (6.03, -44.2642) (6.03, -44.1243) (5.834, -43.9283) (5.6941, -43.9283) knots 0 0 0 1 2 2 2
  line L2410 (6.03, -44.2642) -> (6.03, -44.1243) construction
  line L2411 (6.03, -44.1243) -> (5.834, -43.9283) construction
  line L2412 (5.834, -43.9283) -> (5.6941, -43.9283) construction
  line L2413 (5.6941, -43.9283) -> (5.4101, -43.9283)
  spline S734 degree 2 poles (5.4101, -43.9283) (5.2702, -43.9283) (5.0742, -44.1283) (5.0742, -44.2642) knots 0 0 0 1 2 2 2
  line L2414 (5.4101, -43.9283) -> (5.2702, -43.9283) construction
  line L2415 (5.2702, -43.9283) -> (5.0742, -44.1283) construction
  line L2416 (5.0742, -44.1283) -> (5.0742, -44.2642) construction
  line L2417 (5.0742, -44.2642) -> (5.0742, -45.9838)
  spline S735 degree 2 poles (5.0742, -45.9838) (5.0742, -46.1237) (5.2702, -46.3197) (5.4101, -46.3197) knots 0 0 0 1 2 2 2
  line L2418 (5.0742, -45.9838) -> (5.0742, -46.1237) construction
  line L2419 (5.0742, -46.1237) -> (5.2702, -46.3197) construction
  line L2420 (5.2702, -46.3197) -> (5.4101, -46.3197) construction
  line L2421 (5.4101, -46.3197) -> (5.6941, -46.3197)
  spline S736 degree 2 poles (4.5944, -44.2602) (4.5944, -43.9283) (5.0702, -43.4485) (5.4101, -43.4485) knots 0 0 0 1 2 2 2
  line L2422 (4.5944, -44.2602) -> (4.5944, -43.9283) construction
  line L2423 (4.5944, -43.9283) -> (5.0702, -43.4485) construction
  line L2424 (5.0702, -43.4485) -> (5.4101, -43.4485) construction
  line L2425 (5.4101, -43.4485) -> (5.6941, -43.4485)
  spline S737 degree 2 poles (5.6941, -43.4485) (6.034, -43.4485) (6.5098, -43.9243) (6.5098, -44.2642) knots 0 0 0 1 2 2 2
  line L2426 (5.6941, -43.4485) -> (6.034, -43.4485) construction
  line L2427 (6.034, -43.4485) -> (6.5098, -43.9243) construction
  line L2428 (6.5098, -43.9243) -> (6.5098, -44.2642) construction
  line L2429 (6.5098, -44.2642) -> (6.5098, -45.9838)
  spline S738 degree 2 poles (6.5098, -45.9838) (6.5098, -46.3237) (6.034, -46.7995) (5.6941, -46.7995) knots 0 0 0 1 2 2 2
  line L2430 (6.5098, -45.9838) -> (6.5098, -46.3237) construction
  line L2431 (6.5098, -46.3237) -> (6.034, -46.7995) construction
  line L2432 (6.034, -46.7995) -> (5.6941, -46.7995) construction
  line L2433 (5.6941, -46.7995) -> (5.4101, -46.7995)
  spline S739 degree 2 poles (5.4101, -46.7995) (5.0702, -46.7995) (4.5944, -46.3277) (4.5944, -45.9878) knots 0 0 0 1 2 2 2
  line L2434 (5.4101, -46.7995) -> (5.0702, -46.7995) construction
  line L2435 (5.0702, -46.7995) -> (4.5944, -46.3277) construction
  line L2436 (4.5944, -46.3277) -> (4.5944, -45.9878) construction
  spline S740 degree 2 poles (4.1185, -46.5596) (4.1185, -46.7995) (3.8786, -46.7995) knots 0 0 0 1 1 1
  line L2437 (4.1185, -46.5596) -> (4.1185, -46.7995) construction
  line L2438 (4.1185, -46.7995) -> (3.8786, -46.7995) construction
  spline S741 degree 2 poles (3.8786, -46.7995) (3.6386, -46.7995) (3.6386, -46.5596) knots 0 0 0 1 1 1
  line L2439 (3.8786, -46.7995) -> (3.6386, -46.7995) construction
  line L2440 (3.6386, -46.7995) -> (3.6386, -46.5596) construction
  line L2441 (3.6386, -46.5596) -> (3.6386, -43.6884)
  spline S742 degree 2 poles (3.6386, -43.6884) (3.6386, -43.4485) (3.8786, -43.4485) knots 0 0 0 1 1 1
  line L2442 (3.6386, -43.6884) -> (3.6386, -43.4485) construction
  line L2443 (3.6386, -43.4485) -> (3.8786, -43.4485) construction
  spline S743 degree 2 poles (3.8786, -43.4485) (4.1185, -43.4485) (4.1185, -43.6884) knots 0 0 0 1 1 1
  line L2444 (3.8786, -43.4485) -> (4.1185, -43.4485) construction
  line L2445 (4.1185, -43.4485) -> (4.1185, -43.6884) construction
  spline S744 degree 2 poles (10.3408, -43.6884) (10.3408, -43.4485) (10.5807, -43.4485) knots 0 0 0 1 1 1
  line L2446 (10.3408, -43.6884) -> (10.3408, -43.4485) construction
  line L2447 (10.3408, -43.4485) -> (10.5807, -43.4485) construction
  spline S745 degree 2 poles (10.5807, -43.4485) (10.8206, -43.4485) (10.8206, -43.6884) knots 0 0 0 1 1 1
  line L2448 (10.5807, -43.4485) -> (10.8206, -43.4485) construction
  line L2449 (10.8206, -43.4485) -> (10.8206, -43.6884) construction
  spline S746 degree 2 poles (11.0606, -46.3197) (11.3005, -46.3197) (11.3005, -46.5596) knots 0 0 0 1 1 1
  line L2450 (11.0606, -46.3197) -> (11.3005, -46.3197) construction
  line L2451 (11.3005, -46.3197) -> (11.3005, -46.5596) construction
  line L2452 (11.3005, -46.5596) -> (11.3005, -47.0355)
  spline S747 degree 2 poles (11.3005, -47.0355) (11.3005, -47.2754) (11.0606, -47.2754) knots 0 0 0 1 1 1
  line L2453 (11.3005, -47.0355) -> (11.3005, -47.2754) construction
  line L2454 (11.3005, -47.2754) -> (11.0606, -47.2754) construction
  spline S748 degree 2 poles (11.0606, -47.2754) (10.8206, -47.2754) (10.8206, -47.0355) knots 0 0 0 1 1 1
  line L2455 (11.0606, -47.2754) -> (10.8206, -47.2754) construction
  line L2456 (10.8206, -47.2754) -> (10.8206, -47.0355) construction
  spline S749 degree 2 poles (8.4253, -46.7995) (8.0294, -46.7995) (7.4696, -46.2397) (7.4696, -45.8438) knots 0 0 0 1 2 2 2
  line L2457 (8.4253, -46.7995) -> (8.0294, -46.7995) construction
  line L2458 (8.0294, -46.7995) -> (7.4696, -46.2397) construction
  line L2459 (7.4696, -46.2397) -> (7.4696, -45.8438) construction
  line L2460 (7.4696, -45.8438) -> (7.4696, -43.6884)
  spline S750 degree 2 poles (7.4696, -43.6884) (7.4696, -43.4485) (7.7095, -43.4485) knots 0 0 0 1 1 1
  line L2461 (7.4696, -43.6884) -> (7.4696, -43.4485) construction
  line L2462 (7.4696, -43.4485) -> (7.7095, -43.4485) construction
  spline S751 degree 2 poles (7.7095, -43.4485) (7.9494, -43.4485) (7.9494, -43.6884) knots 0 0 0 1 1 1
  line L2463 (7.7095, -43.4485) -> (7.9494, -43.4485) construction
  line L2464 (7.9494, -43.4485) -> (7.9494, -43.6884) construction
  line L2465 (7.9494, -43.6884) -> (7.9494, -45.8398)
  spline S752 degree 2 poles (7.9494, -45.8398) (7.9494, -46.0357) (8.2333, -46.3197) (8.4293, -46.3197) knots 0 0 0 1 2 2 2
  line L2466 (7.9494, -45.8398) -> (7.9494, -46.0357) construction
  line L2467 (7.9494, -46.0357) -> (8.2333, -46.3197) construction
  line L2468 (8.2333, -46.3197) -> (8.4293, -46.3197) construction
  spline S753 degree 2 poles (8.9052, -43.6884) (8.9052, -43.4485) (9.1451, -43.4485) knots 0 0 0 1 1 1
  line L2469 (8.9052, -43.6884) -> (8.9052, -43.4485) construction